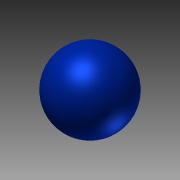
# Autodesk Inventor part: Ball
Saved by Autodesk Inventor 2012 (Build 160160000, 160)
## iProperties
Created: 2012-10-02
Part Number: Ball
Material: Default
Document SubType Name: Modeling
Designer: agmlego
Density: 1 g/cm^3
Author: agmlego
Autodesk Inventor part; units mm, degrees
ref_plane "YZ Plane" through (0, 0, 0) normal (1, 0, 0) x (0, 1, 0)
ref_plane "XZ Plane" through (0, 0, 0) normal (0, 1, 0) x (-1, 0, 0)
ref_plane "XY Plane" through (0, 0, 0) normal (0, 0, 1) x (1, 0, 0)
sketch "Sketch2" plane through (0, 0, 0) normal (0, 0, 1) x (1, 0, 0)
  arc A0 (28.575, 0) -> (-28.575, 0) centre (0, 0) ccw
  line L0 (-28.575, 0) -> (28.575, 0)
  line L1 (-28.575, 0) -> (-28.575, -70.3192) construction
  line L2 (28.575, 0) -> (28.575, -70.3192) construction
  dimension "d0" = 28.575
  constraints: 6 end point, 2 point on circle, 2 tangent, 1 centre point, 1 coincident, 1 horizontal, 1 parallel, 1 perpendicular
  measures "d0" radius of A0
revolve "Revolution1" add sketch "Sketch2" angle 360 about axis through (-28.575, 0, 0) along (1, 0, 0)
body "Solid1"
